Autodesk Inventor part; units mm, degrees
(part 2 of 2)
  arc A252 (-6.9792, -17.505) -> (-6.5266, -17.6787) centre (0, 0) ccw projected
  arc A253 (-6.5266, -17.6787) -> (-6.34, -17.6043) centre (-6.4746, -17.538) ccw projected
  arc A254 (-6.1625, -17.3517) -> (-6.34, -17.6043) centre (-5.443, -18.0463) ccw projected
  arc A255 (-5.2136, -17.6601) -> (-6.1625, -17.3517) centre (-5.7632, -17.7372) ccw projected
  arc A256 (-5.2184, -17.9688) -> (-5.2136, -17.6601) centre (-6.2038, -17.7991) ccw projected
  arc A257 (-5.2184, -17.9688) -> (-5.1112, -18.1386) centre (-5.0705, -17.9942) ccw projected
  arc A258 (-5.1112, -18.1386) -> (-4.6429, -18.2641) centre (0, 0) ccw projected
  arc A259 (-4.6429, -18.2641) -> (-4.4652, -18.1706) centre (-4.6059, -18.1187) ccw projected
  arc A260 (-4.315, -17.9008) -> (-4.4652, -18.1706) centre (-3.5268, -18.5164) ccw projected
  arc A261 (-3.339, -18.1083) -> (-4.315, -17.9008) centre (-3.8776, -18.2425) ccw projected
  arc A262 (-3.3115, -18.4158) -> (-3.339, -18.1083) centre (-4.3094, -18.35) ccw projected
  arc A263 (-3.3115, -18.4158) -> (-3.1872, -18.5735) centre (-3.1618, -18.4257) ccw projected
  arc A264 (-3.1872, -18.5735) -> (-2.7083, -18.6494) centre (0, 0) ccw projected
  arc A265 (-2.7083, -18.6494) -> (-2.5414, -18.5378) centre (-2.6868, -18.5009) ccw projected
  arc A266 (-2.4202, -18.2538) -> (-2.5414, -18.5378) centre (-1.572, -18.7836) ccw projected
  arc A267 (-1.4279, -18.3581) -> (-2.4202, -18.2538) centre (-1.9495, -18.5478) ccw projected
  arc A268 (-1.3684, -18.6611) -> (-1.4279, -18.3581) centre (-2.3676, -18.7) ccw projected
  arc A269 (-1.3684, -18.6611) -> (-1.2283, -18.8049) centre (-1.2185, -18.6552) ccw projected
  arc A270 (-1.2283, -18.8049) -> (-0.7441, -18.8303) centre (0, 0) ccw projected
  arc A271 (-0.7441, -18.8303) -> (-0.5897, -18.7019) centre (-0.7382, -18.6804) ccw projected
  arc A272 (-0.4989, -18.4068) -> (-0.5897, -18.7019) centre (0.4, -18.845) ccw projected
  arc A273 (0.4989, -18.4068) -> (-0.4989, -18.4068) centre (0, -18.65) ccw projected
  arc A274 (0.5897, -18.7019) -> (0.4989, -18.4068) centre (-0.4, -18.845) ccw projected
  arc A275 (0.5897, -18.7019) -> (0.7441, -18.8303) centre (0.7382, -18.6804) ccw projected
  arc A276 (0.7441, -18.8303) -> (1.2283, -18.8049) centre (0, 0) ccw projected
  arc A277 (1.2283, -18.8049) -> (1.3684, -18.6611) centre (1.2185, -18.6552) ccw projected
  arc A278 (1.4279, -18.3581) -> (1.3684, -18.6611) centre (2.3676, -18.7) ccw projected
  arc A279 (2.4202, -18.2538) -> (1.4279, -18.3581) centre (1.9495, -18.5478) ccw projected
  arc A280 (2.5414, -18.5378) -> (2.4202, -18.2538) centre (1.572, -18.7836) ccw projected
  arc A281 (2.5414, -18.5378) -> (2.7083, -18.6494) centre (2.6868, -18.5009) ccw projected
  arc A282 (2.7083, -18.6494) -> (3.1872, -18.5735) centre (0, 0) ccw projected
  arc A283 (3.1872, -18.5735) -> (3.3115, -18.4158) centre (3.1618, -18.4257) ccw projected
  arc A284 (3.339, -18.1083) -> (3.3115, -18.4158) centre (4.3094, -18.35) ccw projected
  arc A285 (4.315, -17.9008) -> (3.339, -18.1083) centre (3.8776, -18.2425) ccw projected
  arc A286 (4.4652, -18.1706) -> (4.315, -17.9008) centre (3.5268, -18.5164) ccw projected
  arc A287 (4.4652, -18.1706) -> (4.6429, -18.2641) centre (4.6059, -18.1187) ccw projected
  arc A288 (4.6429, -18.2641) -> (5.1112, -18.1386) centre (0, 0) ccw projected
  arc A289 (5.1112, -18.1386) -> (5.2184, -17.9688) centre (5.0705, -17.9942) ccw projected
  arc A290 (5.2136, -17.6601) -> (5.2184, -17.9688) centre (6.2038, -17.7991) ccw projected
  arc A291 (6.1625, -17.3517) -> (5.2136, -17.6601) centre (5.7632, -17.7372) ccw projected
  arc A292 (6.34, -17.6043) -> (6.1625, -17.3517) centre (5.443, -18.0463) ccw projected
  arc A293 (6.34, -17.6043) -> (6.5266, -17.6787) centre (6.4746, -17.538) ccw projected
  arc A294 (6.5266, -17.6787) -> (6.9792, -17.505) centre (0, 0) ccw projected
  arc A295 (6.9792, -17.505) -> (7.068, -17.3249) centre (6.9237, -17.3657) ccw projected
  arc A296 (7.031, -17.0184) -> (7.068, -17.3249) centre (8.0304, -17.0531) ccw projected
  arc A297 (7.9425, -16.6125) -> (7.031, -17.0184) centre (7.5856, -17.0376) ccw projected
  arc A298 (8.1455, -16.8452) -> (7.9425, -16.6125) centre (7.2995, -17.3785) ccw projected
  arc A299 (8.1455, -16.8452) -> (8.3387, -16.8997) centre (8.2724, -16.7652) ccw projected
  arc A300 (8.3387, -16.8997) -> (8.7708, -16.6796) centre (0, 0) ccw projected
  arc A301 (8.7708, -16.6796) -> (8.8402, -16.4912) centre (8.7009, -16.5468) ccw projected
  arc A302 (8.7714, -16.1902) -> (8.8402, -16.4912) centre (9.7689, -16.1202) ccw projected
  arc A303 (9.6354, -15.6913) -> (8.7714, -16.1902) centre (9.325, -16.1514) ccw projected
  arc A304 (9.8616, -15.9015) -> (9.6354, -15.6913) centre (9.0761, -16.5202) ccw projected
  arc A305 (9.8616, -15.9015) -> (10.0595, -15.9355) centre (9.9795, -15.8086) ccw projected
  arc A306 (10.0595, -15.9355) -> (10.4662, -15.6714) centre (0, 0) ccw projected
  arc A307 (10.4662, -15.6714) -> (10.5156, -15.4768) centre (10.3829, -15.5467) ccw projected
  arc A308 (10.4156, -15.1846) -> (10.5156, -15.4768) centre (11.4004, -15.0108) ccw projected
  arc A309 (11.2228, -14.5982) -> (10.4156, -15.1846) centre (10.9622, -15.0882) ccw projected
  arc A310 (11.4698, -14.7835) -> (11.2228, -14.5982) centre (10.7532, -15.481) ccw projected
  arc A311 (11.4698, -14.7835) -> (11.6702, -14.7967) centre (11.5773, -14.6789) ccw projected
  arc A312 (11.6702, -14.7967) -> (12.047, -14.4915) centre (0, 0) ccw projected
  arc A313 (12.047, -14.4915) -> (12.0758, -14.2928) centre (11.9511, -14.3762) ccw projected
  arc A314 (11.9458, -14.0127) -> (12.0758, -14.2928) centre (12.907, -13.7369) ccw projected
  arc A315 (12.6873, -13.3451) -> (11.9458, -14.0127) centre (12.4793, -13.8597) ccw projected
  arc A316 (12.9522, -13.5036) -> (12.6873, -13.3451) centre (12.3125, -14.2722) ccw projected
  arc A317 (12.9522, -13.5036) -> (13.1529, -13.4958) centre (13.0482, -13.3883) ccw projected
  arc A318 (13.1529, -13.4958) -> (13.4958, -13.1529) centre (0, 0) ccw projected
  arc A319 (13.4958, -13.1529) -> (13.5036, -12.9522) centre (13.3883, -13.0482) ccw projected
  arc A320 (13.3451, -12.6873) -> (13.5036, -12.9522) centre (14.2722, -12.3125) ccw projected
  arc A321 (14.0127, -11.9458) -> (13.3451, -12.6873) centre (13.8597, -12.4793) ccw projected
  arc A322 (14.2928, -12.0758) -> (14.0127, -11.9458) centre (13.7369, -12.907) ccw projected
  arc A323 (14.2928, -12.0758) -> (14.4915, -12.047) centre (14.3762, -11.9511) ccw projected
  arc A324 (14.4915, -12.047) -> (14.7967, -11.6702) centre (0, 0) ccw projected
  arc A325 (14.7967, -11.6702) -> (14.7835, -11.4698) centre (14.6789, -11.5773) ccw projected
  arc A326 (14.5982, -11.2228) -> (14.7835, -11.4698) centre (15.481, -10.7532) ccw projected
  arc A327 (15.1846, -10.4156) -> (14.5982, -11.2228) centre (15.0882, -10.9622) ccw projected
  arc A328 (15.4768, -10.5156) -> (15.1846, -10.4156) centre (15.0108, -11.4004) ccw projected
  arc A329 (15.4768, -10.5156) -> (15.6714, -10.4662) centre (15.5467, -10.3829) ccw projected
  arc A330 (15.6714, -10.4662) -> (15.9355, -10.0595) centre (0, 0) ccw projected
  arc A331 (15.9355, -10.0595) -> (15.9015, -9.8616) centre (15.8086, -9.9795) ccw projected
  arc A332 (15.6913, -9.6354) -> (15.9015, -9.8616) centre (16.5202, -9.0761) ccw projected
  arc A333 (16.1902, -8.7714) -> (15.6913, -9.6354) centre (16.1514, -9.325) ccw projected
  arc A334 (16.4912, -8.8402) -> (16.1902, -8.7714) centre (16.1202, -9.7689) ccw projected
  arc A335 (16.4912, -8.8402) -> (16.6796, -8.7708) centre (16.5468, -8.7009) ccw projected
  arc A336 (16.6796, -8.7708) -> (16.8997, -8.3387) centre (0, 0) ccw projected
  arc A337 (16.8997, -8.3387) -> (16.8452, -8.1455) centre (16.7652, -8.2724) ccw projected
  arc A338 (16.6125, -7.9425) -> (16.8452, -8.1455) centre (17.3785, -7.2995) ccw projected
  arc A339 (17.0184, -7.031) -> (16.6125, -7.9425) centre (17.0376, -7.5856) ccw projected
  arc A340 (17.3249, -7.068) -> (17.0184, -7.031) centre (17.0531, -8.0304) ccw projected
  arc A341 (17.3249, -7.068) -> (17.505, -6.9792) centre (17.3657, -6.9237) ccw projected
  arc A342 (17.505, -6.9792) -> (17.6787, -6.5266) centre (0, 0) ccw projected
  arc A343 (17.6787, -6.5266) -> (17.6043, -6.34) centre (17.538, -6.4746) ccw projected
  arc A344 (17.3517, -6.1625) -> (17.6043, -6.34) centre (18.0463, -5.443) ccw projected
  arc A345 (17.6601, -5.2136) -> (17.3517, -6.1625) centre (17.7372, -5.7632) ccw projected
  arc A346 (17.9688, -5.2184) -> (17.6601, -5.2136) centre (17.7991, -6.2038) ccw projected
  arc A347 (17.9688, -5.2184) -> (18.1386, -5.1112) centre (17.9942, -5.0705) ccw projected
  arc A348 (18.1386, -5.1112) -> (18.2641, -4.6429) centre (0, 0) ccw projected
  arc A349 (18.2641, -4.6429) -> (18.1706, -4.4652) centre (18.1187, -4.6059) ccw projected
  arc A350 (17.9008, -4.315) -> (18.1706, -4.4652) centre (18.5164, -3.5268) ccw projected
  arc A351 (18.1083, -3.339) -> (17.9008, -4.315) centre (18.2425, -3.8776) ccw projected
  arc A352 (18.4158, -3.3115) -> (18.1083, -3.339) centre (18.35, -4.3094) ccw projected
  arc A353 (18.4158, -3.3115) -> (18.5735, -3.1872) centre (18.4257, -3.1618) ccw projected
  arc A354 (18.5735, -3.1872) -> (18.6494, -2.7083) centre (0, 0) ccw projected
  arc A355 (18.6494, -2.7083) -> (18.5378, -2.5414) centre (18.5009, -2.6868) ccw projected
  arc A356 (18.2538, -2.4202) -> (18.5378, -2.5414) centre (18.7836, -1.572) ccw projected
  arc A357 (18.3581, -1.4279) -> (18.2538, -2.4202) centre (18.5478, -1.9495) ccw projected
  arc A358 (18.6611, -1.3684) -> (18.3581, -1.4279) centre (18.7, -2.3676) ccw projected
  arc A359 (18.6611, -1.3684) -> (18.8049, -1.2283) centre (18.6552, -1.2185) ccw projected
  line L0 (-2, 8.1235) -> (2, 8.1235) projected
  line L1 (2, 8.1235) -> (2, 5.1235) projected
  arc A360 (-2, 5.1235) -> (2, 5.1235) centre (0, 0) ccw projected
  line L2 (-2, 5.1235) -> (-2, 8.1235) projected
